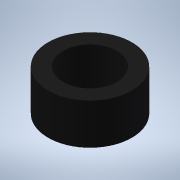
# Autodesk Inventor part: 3
Saved by Autodesk Inventor 2021 (Build 250183000, 183)
## iProperties
Created: 2012-06-12
Part Number: 3
Material: Genérico
Document SubType Name: Modeling
Designer: Luis
Density: 1 g/cm^3
Appearance: Brillante - Negro
Author: Luis
Autodesk Inventor part; units mm, degrees
ref_plane "YZ Plane" through (0, 0, 0) normal (1, 0, 0) x (0, 1, 0)
ref_plane "XZ Plane" through (0, 0, 0) normal (0, 1, 0) x (-1, 0, 0)
ref_plane "XY Plane" through (0, 0, 0) normal (0, 0, 1) x (1, 0, 0)
sketch "Sketch1" plane through (0, 0, 0) normal (0, 0, 1) x (1, 0, 0)
  circle A0 centre (0, 0) radius 21
  circle A1 centre (0, 0) radius 13.5
  dimension "d0" = 42
  dimension "d1" = 7.5
  constraints: 2 centre point, 2 coincident
  measures "d0" diameter of A0
  measures "d1" radial gap between concentric circles of A1 A0
extrude "Extrusion1" add sketch "Sketch1" along normal blind 20.5
body "Solid1"
